Autodesk Inventor part; units mm, degrees
(part 2 of 2)
sketch "Эскиз8" plane through (0, 0, 0) normal (0, -1, 0) x (1, 0, 0)
  line L0 (48.9974, -0.5) -> (48.1, -0.4908) construction
  line L1 (48.1, -0.4908) -> (48.1, -0.85) construction
  arc A0 (46.1, -2.85) -> (48.1, -0.85) centre (46.1, -0.85) ccw construction
  line L2 (46.1, -2.85) -> (42.7, -2.85) construction
  line L3 (42.7, -2.85) -> (42.7, 2.85) construction
  line L4 (42.7, 2.85) -> (46.1, 2.85) construction
  arc A1 (48.1, 0.85) -> (46.1, 2.85) centre (46.1, 0.85) ccw construction
  line L5 (48.1, 0.85) -> (48.1, 0.4908) construction
  line L6 (48.1, 0.4908) -> (48.9974, 0.5) construction
  arc A2 (48.9974, -0.5) -> (48.9974, 0.5) centre (0, 0) ccw construction
  arc A3 (47.9584, -10.0493) -> (48.1535, -9.0685) centre (0, 0) ccw construction
  line L7 (47.9584, -10.0493) -> (47.08, -9.8653) construction
  line L8 (47.08, -9.8653) -> (47.0099, -10.2175) construction
  arc A4 (44.6582, -11.7889) -> (47.0099, -10.2175) centre (45.0484, -9.8273) ccw construction
  line L9 (44.6582, -11.7889) -> (41.3235, -11.1256) construction
  line L10 (41.3235, -11.1256) -> (42.4355, -5.5351) construction
  line L11 (42.4355, -5.5351) -> (45.7702, -6.1984) construction
  arc A5 (47.3416, -8.5502) -> (45.7702, -6.1984) centre (45.38, -8.16) ccw construction
  line L12 (47.3416, -8.5502) -> (47.2715, -8.9024) construction
  line L13 (47.2715, -8.9024) -> (48.1535, -9.0685) construction
  line L14 (48.1535, 9.0685) -> (47.2715, 8.9024) construction
  line L15 (47.2715, 8.9024) -> (47.3416, 8.5502) construction
  arc A6 (45.7702, 6.1984) -> (47.3416, 8.5502) centre (45.38, 8.16) ccw construction
  line L16 (45.7702, 6.1984) -> (42.4355, 5.5351) construction
  line L17 (42.4355, 5.5351) -> (41.3235, 11.1256) construction
  line L18 (41.3235, 11.1256) -> (44.6582, 11.7889) construction
  arc A7 (47.0099, 10.2175) -> (44.6582, 11.7889) centre (45.0484, 9.8273) ccw construction
  line L19 (47.0099, 10.2175) -> (47.08, 9.8653) construction
  line L20 (47.08, 9.8653) -> (47.9584, 10.0493) construction
  arc A8 (48.1535, 9.0685) -> (47.9584, 10.0493) centre (0, 0) ccw construction
  arc A9 (45.0764, -19.2125) -> (45.4591, -18.2886) centre (0, 0) ccw construction
  line L21 (45.0764, -19.2125) -> (44.2508, -18.8606) construction
  line L22 (44.2508, -18.8606) -> (44.1133, -19.1924) construction
  arc A10 (41.5002, -20.2748) -> (44.1133, -19.1924) centre (42.2656, -18.427) ccw construction
  line L23 (41.5002, -20.2748) -> (38.359, -18.9736) construction
  line L24 (38.359, -18.9736) -> (40.5403, -13.7075) construction
  line L25 (40.5403, -13.7075) -> (43.6815, -15.0086) construction
  arc A11 (44.7639, -17.6218) -> (43.6815, -15.0086) centre (42.9161, -16.8564) ccw construction
  line L26 (44.7639, -17.6218) -> (44.6264, -17.9536) construction
  line L27 (44.6264, -17.9536) -> (45.4591, -18.2886) construction
  line L28 (45.4591, 18.2886) -> (44.6264, 17.9536) construction
  line L29 (44.6264, 17.9536) -> (44.7639, 17.6218) construction
  arc A12 (43.6815, 15.0086) -> (44.7639, 17.6218) centre (42.9161, 16.8564) ccw construction
  line L30 (43.6815, 15.0086) -> (40.5403, 13.7075) construction
  line L31 (40.5403, 13.7075) -> (38.359, 18.9736) construction
  line L32 (38.359, 18.9736) -> (41.5002, 20.2748) construction
  arc A13 (44.1133, 19.1924) -> (41.5002, 20.2748) centre (42.2656, 18.427) ccw construction
  line L33 (44.1133, 19.1924) -> (44.2508, 18.8606) construction
  line L34 (44.2508, 18.8606) -> (45.0764, 19.2125) construction
  arc A14 (45.4591, 18.2886) -> (45.0764, 19.2125) centre (0, 0) ccw construction
  arc A15 (40.4621, -27.6373) -> (41.0177, -26.8058) centre (0, 0) ccw construction
  line L35 (40.4621, -27.6373) -> (39.721, -27.131) construction
  line L36 (39.721, -27.131) -> (39.5215, -27.4297) construction
  arc A16 (36.7474, -27.9815) -> (39.5215, -27.4297) centre (37.8585, -26.3185) ccw construction
  line L37 (36.7474, -27.9815) -> (33.9204, -26.0925) construction
  line L38 (33.9204, -26.0925) -> (37.0871, -21.3532) construction
  line L39 (37.0871, -21.3532) -> (39.9141, -23.2421) construction
  arc A17 (40.4659, -26.0162) -> (39.9141, -23.2421) centre (38.803, -24.905) ccw construction
  line L40 (40.4659, -26.0162) -> (40.2664, -26.3148) construction
  line L41 (40.2664, -26.3148) -> (41.0177, -26.8058) construction
  line L42 (41.0177, 26.8058) -> (40.2664, 26.3148) construction
  line L43 (40.2664, 26.3148) -> (40.4659, 26.0162) construction
  arc A18 (39.9141, 23.2421) -> (40.4659, 26.0162) centre (38.803, 24.905) ccw construction
  line L44 (39.9141, 23.2421) -> (37.0871, 21.3532) construction
  line L45 (37.0871, 21.3532) -> (33.9204, 26.0925) construction
  line L46 (33.9204, 26.0925) -> (36.7474, 27.9815) construction
  arc A19 (39.5215, 27.4297) -> (36.7474, 27.9815) centre (37.8585, 26.3185) ccw construction
  line L47 (39.5215, 27.4297) -> (39.721, 27.131) construction
  line L48 (39.721, 27.131) -> (40.4621, 27.6373) construction
  arc A20 (41.0177, 26.8058) -> (40.4621, 27.6373) centre (0, 0) ccw construction
  arc A21 (34.2929, -35) -> (35, -34.2929) centre (0, 0) ccw construction
  line L49 (34.2929, -35) -> (33.6648, -34.3589) construction
  line L50 (33.6648, -34.3589) -> (33.4108, -34.6129) construction
  arc A22 (30.5824, -34.6129) -> (33.4108, -34.6129) centre (31.9966, -33.1987) ccw construction
  line L51 (30.5824, -34.6129) -> (28.1782, -32.2087) construction
  line L52 (28.1782, -32.2087) -> (32.2087, -28.1782) construction
  line L53 (32.2087, -28.1782) -> (34.6129, -30.5824) construction
  arc A23 (34.6129, -33.4108) -> (34.6129, -30.5824) centre (33.1987, -31.9966) ccw construction
  line L54 (34.6129, -33.4108) -> (34.3589, -33.6648) construction
  line L55 (34.3589, -33.6648) -> (35, -34.2929) construction
  line L56 (35, 34.2929) -> (34.3589, 33.6648) construction
  line L57 (34.3589, 33.6648) -> (34.6129, 33.4108) construction
  arc A24 (34.6129, 30.5824) -> (34.6129, 33.4108) centre (33.1987, 31.9966) ccw construction
  line L58 (34.6129, 30.5824) -> (32.2087, 28.1782) construction
  line L59 (32.2087, 28.1782) -> (28.1782, 32.2087) construction
  line L60 (28.1782, 32.2087) -> (30.5824, 34.6129) construction
  arc A25 (33.4108, 34.6129) -> (30.5824, 34.6129) centre (31.9966, 33.1987) ccw construction
  line L61 (33.4108, 34.6129) -> (33.6648, 34.3589) construction
  line L62 (33.6648, 34.3589) -> (34.2929, 35) construction
  arc A26 (35, 34.2929) -> (34.2929, 35) centre (0, 0) ccw construction
  arc A27 (26.8058, -41.0177) -> (27.6373, -40.4621) centre (0, 0) ccw construction
  line L63 (26.8058, -41.0177) -> (26.3148, -40.2664) construction
  line L64 (26.3148, -40.2664) -> (26.0162, -40.4659) construction
  arc A28 (23.2421, -39.9141) -> (26.0162, -40.4659) centre (24.905, -38.803) ccw construction
  line L65 (23.2421, -39.9141) -> (21.3532, -37.0871) construction
  line L66 (21.3532, -37.0871) -> (26.0925, -33.9204) construction
  line L67 (26.0925, -33.9204) -> (27.9815, -36.7474) construction
  arc A29 (27.4297, -39.5215) -> (27.9815, -36.7474) centre (26.3185, -37.8585) ccw construction
  line L68 (27.4297, -39.5215) -> (27.131, -39.721) construction
  line L69 (27.131, -39.721) -> (27.6373, -40.4621) construction
  line L70 (27.6373, 40.4621) -> (27.131, 39.721) construction
  line L71 (27.131, 39.721) -> (27.4297, 39.5215) construction
  arc A30 (27.9815, 36.7474) -> (27.4297, 39.5215) centre (26.3185, 37.8585) ccw construction
  line L72 (27.9815, 36.7474) -> (26.0925, 33.9204) construction
  line L73 (26.0925, 33.9204) -> (21.3532, 37.0871) construction
  line L74 (21.3532, 37.0871) -> (23.2421, 39.9141) construction
  arc A31 (26.0162, 40.4659) -> (23.2421, 39.9141) centre (24.905, 38.803) ccw construction
  line L75 (26.0162, 40.4659) -> (26.3148, 40.2664) construction
  line L76 (26.3148, 40.2664) -> (26.8058, 41.0177) construction
  arc A32 (27.6373, 40.4621) -> (26.8058, 41.0177) centre (0, 0) ccw construction
  arc A33 (18.2886, -45.4591) -> (19.2125, -45.0764) centre (0, 0) ccw construction
  line L77 (18.2886, -45.4591) -> (17.9536, -44.6264) construction
  line L78 (17.9536, -44.6264) -> (17.6218, -44.7639) construction
  arc A34 (15.0086, -43.6815) -> (17.6218, -44.7639) centre (16.8564, -42.9161) ccw construction
  line L79 (15.0086, -43.6815) -> (13.7075, -40.5403) construction
  line L80 (13.7075, -40.5403) -> (18.9736, -38.359) construction
  line L81 (18.9736, -38.359) -> (20.2748, -41.5002) construction
  arc A35 (19.1924, -44.1133) -> (20.2748, -41.5002) centre (18.427, -42.2656) ccw construction
  line L82 (19.1924, -44.1133) -> (18.8606, -44.2508) construction
  line L83 (18.8606, -44.2508) -> (19.2125, -45.0764) construction
  line L84 (19.2125, 45.0764) -> (18.8606, 44.2508) construction
  line L85 (18.8606, 44.2508) -> (19.1924, 44.1133) construction
  arc A36 (20.2748, 41.5002) -> (19.1924, 44.1133) centre (18.427, 42.2656) ccw construction
  line L86 (20.2748, 41.5002) -> (18.9736, 38.359) construction
  line L87 (18.9736, 38.359) -> (13.7075, 40.5403) construction
  line L88 (13.7075, 40.5403) -> (15.0086, 43.6815) construction
  arc A37 (17.6218, 44.7639) -> (15.0086, 43.6815) centre (16.8564, 42.9161) ccw construction
  line L89 (17.6218, 44.7639) -> (17.9536, 44.6264) construction
  line L90 (17.9536, 44.6264) -> (18.2886, 45.4591) construction
  arc A38 (19.2125, 45.0764) -> (18.2886, 45.4591) centre (0, 0) ccw construction
  arc A39 (9.0685, -48.1535) -> (10.0493, -47.9584) centre (0, 0) ccw construction
  line L91 (9.0685, -48.1535) -> (8.9024, -47.2715) construction
  line L92 (8.9024, -47.2715) -> (8.5502, -47.3416) construction
  arc A40 (6.1984, -45.7702) -> (8.5502, -47.3416) centre (8.16, -45.38) ccw construction
  line L93 (6.1984, -45.7702) -> (5.5351, -42.4355) construction
  line L94 (5.5351, -42.4355) -> (11.1256, -41.3235) construction
  line L95 (11.1256, -41.3235) -> (11.7889, -44.6582) construction
  arc A41 (10.2175, -47.0099) -> (11.7889, -44.6582) centre (9.8273, -45.0484) ccw construction
  line L96 (10.2175, -47.0099) -> (9.8653, -47.08) construction
  line L97 (9.8653, -47.08) -> (10.0493, -47.9584) construction
  line L98 (10.0493, 47.9584) -> (9.8653, 47.08) construction
  line L99 (9.8653, 47.08) -> (10.2175, 47.0099) construction
  arc A42 (11.7889, 44.6582) -> (10.2175, 47.0099) centre (9.8273, 45.0484) ccw construction
  line L100 (11.7889, 44.6582) -> (11.1256, 41.3235) construction
  line L101 (11.1256, 41.3235) -> (5.5351, 42.4355) construction
  line L102 (5.5351, 42.4355) -> (6.1984, 45.7702) construction
  arc A43 (8.5502, 47.3416) -> (6.1984, 45.7702) centre (8.16, 45.38) ccw construction
  line L103 (8.5502, 47.3416) -> (8.9024, 47.2715) construction
  line L104 (8.9024, 47.2715) -> (9.0685, 48.1535) construction
  arc A44 (10.0493, 47.9584) -> (9.0685, 48.1535) centre (0, 0) ccw construction
  arc A45 (-0.5, -48.9974) -> (0.5, -48.9974) centre (0, 0) ccw projected
  line L105 (-0.5, -48.9974) -> (-0.4908, -48.1) construction
  line L106 (-0.4908, -48.1) -> (-0.85, -48.1) construction
  arc A46 (-2.85, -46.1) -> (-0.85, -48.1) centre (-0.85, -46.1) ccw construction
  line L107 (-2.85, -46.1) -> (-2.85, -42.7) construction
  line L108 (-2.85, -42.7) -> (2.85, -42.7) construction
  line L109 (2.85, -42.7) -> (2.85, -46.1) construction
  arc A47 (0.85, -48.1) -> (2.85, -46.1) centre (0.85, -46.1) ccw construction
  line L110 (0.85, -48.1) -> (0.4908, -48.1) construction
  line L111 (0.4908, -48.1) -> (0.5, -48.9974) construction
  line L112 (0.5, 48.9974) -> (0.4908, 48.1) construction
  line L113 (0.4908, 48.1) -> (0.85, 48.1) construction
  arc A48 (2.85, 46.1) -> (0.85, 48.1) centre (0.85, 46.1) ccw construction
  line L114 (2.85, 46.1) -> (2.85, 42.7) construction
  line L115 (2.85, 42.7) -> (-2.85, 42.7) construction
  line L116 (-2.85, 42.7) -> (-2.85, 46.1) construction
  arc A49 (-0.85, 48.1) -> (-2.85, 46.1) centre (-0.85, 46.1) ccw construction
  line L117 (-0.85, 48.1) -> (-0.4908, 48.1) construction
  line L118 (-0.4908, 48.1) -> (-0.5, 48.9974) construction
  arc A50 (0.5, 48.9974) -> (-0.5, 48.9974) centre (0, 0) ccw construction
  arc A51 (-10.0493, -47.9584) -> (-9.0685, -48.1535) centre (0, 0) ccw construction
  line L119 (-10.0493, -47.9584) -> (-9.8653, -47.08) construction
  line L120 (-9.8653, -47.08) -> (-10.2175, -47.0099) construction
  arc A52 (-11.7889, -44.6582) -> (-10.2175, -47.0099) centre (-9.8273, -45.0484) ccw construction
  line L121 (-11.7889, -44.6582) -> (-11.1256, -41.3235) construction
  line L122 (-11.1256, -41.3235) -> (-5.5351, -42.4355) construction
  line L123 (-5.5351, -42.4355) -> (-6.1984, -45.7702) construction
  arc A53 (-8.5502, -47.3416) -> (-6.1984, -45.7702) centre (-8.16, -45.38) ccw construction
  line L124 (-8.5502, -47.3416) -> (-8.9024, -47.2715) construction
  line L125 (-8.9024, -47.2715) -> (-9.0685, -48.1535) construction
  line L126 (-9.0685, 48.1535) -> (-8.9024, 47.2715) construction
  line L127 (-8.9024, 47.2715) -> (-8.5502, 47.3416) construction
  arc A54 (-6.1984, 45.7702) -> (-8.5502, 47.3416) centre (-8.16, 45.38) ccw construction
  line L128 (-6.1984, 45.7702) -> (-5.5351, 42.4355) construction
  line L129 (-5.5351, 42.4355) -> (-11.1256, 41.3235) construction
  line L130 (-11.1256, 41.3235) -> (-11.7889, 44.6582) construction
  arc A55 (-10.2175, 47.0099) -> (-11.7889, 44.6582) centre (-9.8273, 45.0484) ccw construction
  line L131 (-10.2175, 47.0099) -> (-9.8653, 47.08) construction
  line L132 (-9.8653, 47.08) -> (-10.0493, 47.9584) construction
  arc A56 (-9.0685, 48.1535) -> (-10.0493, 47.9584) centre (0, 0) ccw construction
  arc A57 (-19.2125, -45.0764) -> (-18.2886, -45.4591) centre (0, 0) ccw construction
  line L133 (-19.2125, -45.0764) -> (-18.8606, -44.2508) construction
  line L134 (-18.8606, -44.2508) -> (-19.1924, -44.1133) construction
  arc A58 (-20.2748, -41.5002) -> (-19.1924, -44.1133) centre (-18.427, -42.2656) ccw construction
  line L135 (-20.2748, -41.5002) -> (-18.9736, -38.359) construction
  line L136 (-18.9736, -38.359) -> (-13.7075, -40.5403) construction
  line L137 (-13.7075, -40.5403) -> (-15.0086, -43.6815) construction
  arc A59 (-17.6218, -44.7639) -> (-15.0086, -43.6815) centre (-16.8564, -42.9161) ccw construction
  line L138 (-17.6218, -44.7639) -> (-17.9536, -44.6264) construction
  line L139 (-17.9536, -44.6264) -> (-18.2886, -45.4591) construction
  line L140 (-18.2886, 45.4591) -> (-17.9536, 44.6264) construction
  line L141 (-17.9536, 44.6264) -> (-17.6218, 44.7639) construction
  arc A60 (-15.0086, 43.6815) -> (-17.6218, 44.7639) centre (-16.8564, 42.9161) ccw construction
  line L142 (-15.0086, 43.6815) -> (-13.7075, 40.5403) construction
  line L143 (-13.7075, 40.5403) -> (-18.9736, 38.359) construction
  line L144 (-18.9736, 38.359) -> (-20.2748, 41.5002) construction
  arc A61 (-19.1924, 44.1133) -> (-20.2748, 41.5002) centre (-18.427, 42.2656) ccw construction
  line L145 (-19.1924, 44.1133) -> (-18.8606, 44.2508) construction
  line L146 (-18.8606, 44.2508) -> (-19.2125, 45.0764) construction
  arc A62 (-18.2886, 45.4591) -> (-19.2125, 45.0764) centre (0, 0) ccw construction
  arc A63 (-27.6373, -40.4621) -> (-26.8058, -41.0177) centre (0, 0) ccw construction
  line L147 (-27.6373, -40.4621) -> (-27.131, -39.721) construction
  line L148 (-27.131, -39.721) -> (-27.4297, -39.5215) construction
  arc A64 (-27.9815, -36.7474) -> (-27.4297, -39.5215) centre (-26.3185, -37.8585) ccw construction
  line L149 (-27.9815, -36.7474) -> (-26.0925, -33.9204) construction
  line L150 (-26.0925, -33.9204) -> (-21.3532, -37.0871) construction
  line L151 (-21.3532, -37.0871) -> (-23.2421, -39.9141) construction
  arc A65 (-26.0162, -40.4659) -> (-23.2421, -39.9141) centre (-24.905, -38.803) ccw construction
  line L152 (-26.0162, -40.4659) -> (-26.3148, -40.2664) construction
  line L153 (-26.3148, -40.2664) -> (-26.8058, -41.0177) construction
  line L154 (-26.8058, 41.0177) -> (-26.3148, 40.2664) construction
  line L155 (-26.3148, 40.2664) -> (-26.0162, 40.4659) construction
  arc A66 (-23.2421, 39.9141) -> (-26.0162, 40.4659) centre (-24.905, 38.803) ccw construction
  line L156 (-23.2421, 39.9141) -> (-21.3532, 37.0871) construction
  line L157 (-21.3532, 37.0871) -> (-26.0925, 33.9204) construction
  line L158 (-26.0925, 33.9204) -> (-27.9815, 36.7474) construction
  arc A67 (-27.4297, 39.5215) -> (-27.9815, 36.7474) centre (-26.3185, 37.8585) ccw construction
  line L159 (-27.4297, 39.5215) -> (-27.131, 39.721) construction
  line L160 (-27.131, 39.721) -> (-27.6373, 40.4621) construction
  arc A68 (-26.8058, 41.0177) -> (-27.6373, 40.4621) centre (0, 0) ccw construction
  arc A69 (-35, -34.2929) -> (-34.2929, -35) centre (0, 0) ccw construction
  line L161 (-35, -34.2929) -> (-34.3589, -33.6648) construction
  line L162 (-34.3589, -33.6648) -> (-34.6129, -33.4108) construction
  arc A70 (-34.6129, -30.5824) -> (-34.6129, -33.4108) centre (-33.1987, -31.9966) ccw construction
  line L163 (-34.6129, -30.5824) -> (-32.2087, -28.1782) construction
  line L164 (-32.2087, -28.1782) -> (-28.1782, -32.2087) construction
  line L165 (-28.1782, -32.2087) -> (-30.5824, -34.6129) construction
  arc A71 (-33.4108, -34.6129) -> (-30.5824, -34.6129) centre (-31.9966, -33.1987) ccw construction
  line L166 (-33.4108, -34.6129) -> (-33.6648, -34.3589) construction
  line L167 (-33.6648, -34.3589) -> (-34.2929, -35) construction
  line L168 (-34.2929, 35) -> (-33.6648, 34.3589) construction
  line L169 (-33.6648, 34.3589) -> (-33.4108, 34.6129) construction
  arc A72 (-30.5824, 34.6129) -> (-33.4108, 34.6129) centre (-31.9966, 33.1987) ccw construction
  line L170 (-30.5824, 34.6129) -> (-28.1782, 32.2087) construction
  line L171 (-28.1782, 32.2087) -> (-32.2087, 28.1782) construction
  line L172 (-32.2087, 28.1782) -> (-34.6129, 30.5824) construction
  arc A73 (-34.6129, 33.4108) -> (-34.6129, 30.5824) centre (-33.1987, 31.9966) ccw construction
  line L173 (-34.6129, 33.4108) -> (-34.3589, 33.6648) construction
  line L174 (-34.3589, 33.6648) -> (-35, 34.2929) construction
  arc A74 (-34.2929, 35) -> (-35, 34.2929) centre (0, 0) ccw construction
  arc A75 (-41.0177, -26.8058) -> (-40.4621, -27.6373) centre (0, 0) ccw construction
  line L175 (-41.0177, -26.8058) -> (-40.2664, -26.3148) construction
  line L176 (-40.2664, -26.3148) -> (-40.4659, -26.0162) construction
  arc A76 (-39.9141, -23.2421) -> (-40.4659, -26.0162) centre (-38.803, -24.905) ccw construction
  line L177 (-39.9141, -23.2421) -> (-37.0871, -21.3532) construction
  line L178 (-37.0871, -21.3532) -> (-33.9204, -26.0925) construction
  line L179 (-33.9204, -26.0925) -> (-36.7474, -27.9815) construction
  arc A77 (-39.5215, -27.4297) -> (-36.7474, -27.9815) centre (-37.8585, -26.3185) ccw construction
  line L180 (-39.5215, -27.4297) -> (-39.721, -27.131) construction
  line L181 (-39.721, -27.131) -> (-40.4621, -27.6373) construction
  line L182 (-40.4621, 27.6373) -> (-39.721, 27.131) construction
  line L183 (-39.721, 27.131) -> (-39.5215, 27.4297) construction
  arc A78 (-36.7474, 27.9815) -> (-39.5215, 27.4297) centre (-37.8585, 26.3185) ccw construction
  line L184 (-36.7474, 27.9815) -> (-33.9204, 26.0925) construction
  line L185 (-33.9204, 26.0925) -> (-37.0871, 21.3532) construction
  line L186 (-37.0871, 21.3532) -> (-39.9141, 23.2421) construction
  arc A79 (-40.4659, 26.0162) -> (-39.9141, 23.2421) centre (-38.803, 24.905) ccw construction
  line L187 (-40.4659, 26.0162) -> (-40.2664, 26.3148) construction
  line L188 (-40.2664, 26.3148) -> (-41.0177, 26.8058) construction
  arc A80 (-40.4621, 27.6373) -> (-41.0177, 26.8058) centre (0, 0) ccw construction
  arc A81 (-45.4591, -18.2886) -> (-45.0764, -19.2125) centre (0, 0) ccw construction
  line L189 (-45.4591, -18.2886) -> (-44.6264, -17.9536) construction
  line L190 (-44.6264, -17.9536) -> (-44.7639, -17.6218) construction
  arc A82 (-43.6815, -15.0086) -> (-44.7639, -17.6218) centre (-42.9161, -16.8564) ccw construction
  line L191 (-43.6815, -15.0086) -> (-40.5403, -13.7075) construction
  line L192 (-40.5403, -13.7075) -> (-38.359, -18.9736) construction
  line L193 (-38.359, -18.9736) -> (-41.5002, -20.2748) construction
  arc A83 (-44.1133, -19.1924) -> (-41.5002, -20.2748) centre (-42.2656, -18.427) ccw construction
  line L194 (-44.1133, -19.1924) -> (-44.2508, -18.8606) construction
  line L195 (-44.2508, -18.8606) -> (-45.0764, -19.2125) construction
  line L196 (-45.0764, 19.2125) -> (-44.2508, 18.8606) construction
  line L197 (-44.2508, 18.8606) -> (-44.1133, 19.1924) construction
  arc A84 (-41.5002, 20.2748) -> (-44.1133, 19.1924) centre (-42.2656, 18.427) ccw construction
  line L198 (-41.5002, 20.2748) -> (-38.359, 18.9736) construction
  line L199 (-38.359, 18.9736) -> (-40.5403, 13.7075) construction
  line L200 (-40.5403, 13.7075) -> (-43.6815, 15.0086) construction
  arc A85 (-44.7639, 17.6218) -> (-43.6815, 15.0086) centre (-42.9161, 16.8564) ccw construction
  line L201 (-44.7639, 17.6218) -> (-44.6264, 17.9536) construction
  line L202 (-44.6264, 17.9536) -> (-45.4591, 18.2886) construction
  arc A86 (-45.0764, 19.2125) -> (-45.4591, 18.2886) centre (0, 0) ccw construction
  arc A87 (-48.1535, -9.0685) -> (-47.9584, -10.0493) centre (0, 0) ccw construction
  line L203 (-48.1535, -9.0685) -> (-47.2715, -8.9024) construction
  line L204 (-47.2715, -8.9024) -> (-47.3416, -8.5502) construction
  arc A88 (-45.7702, -6.1984) -> (-47.3416, -8.5502) centre (-45.38, -8.16) ccw construction
  line L205 (-45.7702, -6.1984) -> (-42.4355, -5.5351) construction
  line L206 (-42.4355, -5.5351) -> (-41.3235, -11.1256) construction
  line L207 (-41.3235, -11.1256) -> (-44.6582, -11.7889) construction
  arc A89 (-47.0099, -10.2175) -> (-44.6582, -11.7889) centre (-45.0484, -9.8273) ccw construction
  line L208 (-47.0099, -10.2175) -> (-47.08, -9.8653) construction
  line L209 (-47.08, -9.8653) -> (-47.9584, -10.0493) construction
  line L210 (-47.9584, 10.0493) -> (-47.08, 9.8653) construction
  line L211 (-47.08, 9.8653) -> (-47.0099, 10.2175) construction
  arc A90 (-44.6582, 11.7889) -> (-47.0099, 10.2175) centre (-45.0484, 9.8273) ccw construction
  line L212 (-44.6582, 11.7889) -> (-41.3235, 11.1256) construction
  line L213 (-41.3235, 11.1256) -> (-42.4355, 5.5351) construction
  line L214 (-42.4355, 5.5351) -> (-45.7702, 6.1984) construction
  arc A91 (-47.3416, 8.5502) -> (-45.7702, 6.1984) centre (-45.38, 8.16) ccw construction
  line L215 (-47.3416, 8.5502) -> (-47.2715, 8.9024) construction
  line L216 (-47.2715, 8.9024) -> (-48.1535, 9.0685) construction
  arc A92 (-47.9584, 10.0493) -> (-48.1535, 9.0685) centre (0, 0) ccw construction
  circle A93 centre (0, 0) radius 50 construction
  arc A94 (-31.9075, -27.3113) -> (-27.3113, -31.9075) centre (0, 0) ccw construction
  line L217 (-31.482, -26.8858) -> (-31.9075, -27.3113) construction
  arc A95 (-31.482, 26.8858) -> (-31.482, -26.8858) centre (0, 0) ccw construction
  line L218 (-31.9075, 27.3113) -> (-31.482, 26.8858) construction
  arc A96 (-27.3113, 31.9075) -> (-31.9075, 27.3113) centre (0, 0) ccw construction
  line L219 (-26.8858, 31.482) -> (-27.3113, 31.9075) construction
  arc A97 (26.8858, 31.482) -> (-26.8858, 31.482) centre (0, 0) ccw construction
  line L220 (27.3113, 31.9075) -> (26.8858, 31.482) construction
  arc A98 (31.9075, 27.3113) -> (27.3113, 31.9075) centre (0, 0) ccw construction
  line L221 (31.482, 26.8858) -> (31.9075, 27.3113) construction
  arc A99 (31.482, -26.8858) -> (31.482, 26.8858) centre (0, 0) ccw construction
  line L222 (31.9075, -27.3113) -> (31.482, -26.8858) construction
  arc A100 (27.3113, -31.9075) -> (31.9075, -27.3113) centre (0, 0) ccw construction
  line L223 (26.8858, -31.482) -> (27.3113, -31.9075) construction
  arc A101 (-26.8858, -31.482) -> (26.8858, -31.482) centre (0, 0) ccw construction
  line L224 (-27.3113, -31.9075) -> (-26.8858, -31.482) construction
  arc A102 (-48.9974, 0.5) -> (-48.9974, -0.5) centre (0, 0) ccw construction
  line L225 (-48.9974, 0.5) -> (-48.1, 0.4908) construction
  line L226 (-48.1, 0.4908) -> (-48.1, 0.85) construction
  arc A103 (-46.1, 2.85) -> (-48.1, 0.85) centre (-46.1, 0.85) ccw construction
  line L227 (-46.1, 2.85) -> (-42.7, 2.85) construction
  line L228 (-42.7, 2.85) -> (-42.7, -2.85) construction
  line L229 (-42.7, -2.85) -> (-46.1, -2.85) construction
  arc A104 (-48.1, -0.85) -> (-46.1, -2.85) centre (-46.1, -0.85) ccw construction
  line L230 (-48.1, -0.85) -> (-48.1, -0.4908) construction
  line L231 (-48.1, -0.4908) -> (-48.9974, -0.5) construction
  arc A105 (-0.5, -48.9974) -> (0.5, -48.9974) centre (0, 0) ccw construction
  line L232 (-0.5, -48.9974) -> (-0.5, -49.9975)
  circle A106 centre (0, 0) radius 50 construction
  line L233 (0, -42.7) -> (0, -50) construction
  line L234 (0.5, -48.9974) -> (0.5, -49.9975)
  line L235 (-0.5, -49.9975) -> (-0.2434, -50.3901)
  line L236 (-0.2434, -50.3901) -> (0.5, -49.9975)
  constraints: 10 end point, 2 point on circle, 2 vertical, 1 midpoint, 1 symmetric about line
extrude "Выдавливание9" cut sketch "Эскиз8" against normal blind 8
pattern_circular "Круговой массив5" count 32 over 360 about axis through (0, 11, 0) along (0, -1, 0) of "Выдавливание9"
fillet "Сопряжение4" radius 2 1 edges at (-50, 11, 0)
